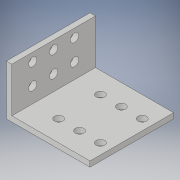
# Autodesk Inventor part: 2in bracket
Saved by Autodesk Inventor 2018 (Build 220112000, 112)
## iProperties
Created: 2020-01-25
Part Number: 2in bracket
Material: Generic
Document SubType Name: Modeling
Designer: s-2513225
Density: 1 g/cm^3
Appearance: Default
Author: s-2513225
Autodesk Inventor part; units mm, degrees
ref_plane "YZ Plane" through (0, 0, 0) normal (1, 0, 0) x (0, 1, 0)
ref_plane "XZ Plane" through (0, 0, 0) normal (0, 1, 0) x (-1, 0, 0)
ref_plane "XY Plane" through (0, 0, 0) normal (0, 0, 1) x (1, 0, 0)
sketch "Sketch1" plane through (0, 0, 0) normal (0, 0, 1) x (1, 0, 0)
  line L0 (0, 0) -> (50.8, 0)
  line L1 (50.8, 0) -> (50.8, 3.302)
  line L2 (50.8, 3.302) -> (3.302, 3.302)
  line L3 (0, 3.302) -> (0, 0)
  line L4 (3.302, 3.302) -> (3.302, 50.8)
  line L5 (3.302, 50.8) -> (0, 50.8)
  line L6 (0, 50.8) -> (0, 3.302)
  dimension "d1" = 3.302
  dimension "d2" = 3.302
  constraints: 14 end point, 3 parallel, 1 horizontal, 1 perpendicular
  measures "d1" distance of L1.end L0.end
  measures "d2" distance of L5.end L4.end
extrude "Extrusion1" add sketch "Sketch1" along normal blind 50.8
sketch "Sketch2" plane through (0, 0, 50.8) normal (0, 0, 1) x (1, 0, 0)
  line L0 (3.302, 50.8) -> (0, 50.8) construction
  line L1 (0, 50.8) -> (0, 30.48) construction
  line L2 (0, 50.8) -> (0, 0) construction
  line L3 (0, 30.48) -> (6.2781, 30.48)
  line L4 (6.2781, 30.48) -> (6.2781, 52.9453)
  line L5 (6.2781, 52.9453) -> (0, 52.9453)
  line L6 (0, 52.9453) -> (0, 30.48)
  line L7 (3.302, 3.302) -> (3.302, 50.8) construction
  line L8 (3.302, 30.48) -> (3.302, 0) construction
  dimension "d6" = 20.32
  dimension "d49" = 30.48
  constraints: 12 end point, 3 point on line, 2 parallel, 1 collinear, 1 horizontal, 1 perpendicular
  measures "d6" distance of L0.end L1.end
  measures "d49" distance of L8.start L8.end
extrude "Extrusion2" cut sketch "Sketch2" against normal blind 50.8
sketch "Sketch3" plane through (0, 0, 0) normal (-1, 0, 0) x (0, 0, 1)
  line L0 (0, 0) -> (50.8, 0) construction
  line L1 (0, 0) -> (12.7, 0) construction
  line L2 (12.7, 0) -> (25.4, 0) construction
  line L3 (25.4, 0) -> (38.1, 0) construction
  line L4 (38.1, 0) -> (38.1, 12.7) construction
  line L5 (38.1, 12.7) -> (38.1, 25.4) construction
  line L6 (25.4, 0) -> (25.4, 12.7) construction
  line L7 (25.4, 12.7) -> (25.4, 25.4) construction
  line L8 (12.7, 0) -> (12.7, 12.7) construction
  line L9 (12.7, 12.7) -> (12.7, 25.4) construction
  circle A0 centre (12.7, 25.4) radius 2.5797
  circle A1 centre (25.4, 25.4) radius 2.5797
  circle A2 centre (38.1, 25.4) radius 2.5797
  circle A3 centre (38.1, 12.7) radius 2.5797
  circle A4 centre (25.4, 12.7) radius 2.5797
  circle A5 centre (12.7, 12.7) radius 2.5797
  dimension "d9" = 12.7
  dimension "d10" = 12.7
  dimension "d11" = 12.7
  dimension "d12" = 12.7
  dimension "d13" = 12.7
  dimension "d14" = 12.7
  dimension "d15" = 12.7
  dimension "d16" = 12.7
  dimension "d17" = 12.7
  dimension "d18" = 5.1594
  dimension "d19" = 5.1594
  dimension "d20" = 5.1594
  dimension "d21" = 5.1594
  dimension "d22" = 5.1594
  dimension "d23" = 5.1594
  constraints: 18 end point, 6 centre point, 6 coincident, 5 point on line, 3 perpendicular, 1 midpoint
  measures "d9" distance of L0.start L1.end
  measures "d10" distance of L1.end L2.end
  measures "d11" distance of L2.end L3.end
  measures "d12" distance of L3.end L4.end
  measures "d13" distance of L4.end L5.end
  measures "d14" distance of L2.end L6.end
  measures "d15" distance of L6.end L7.end
  measures "d16" distance of L1.end L8.end
  measures "d17" distance of L8.end L9.end
  measures "d18" diameter of A0
  measures "d19" diameter of A1
  measures "d20" diameter of A2
  measures "d21" diameter of A3
  measures "d22" diameter of A4
  measures "d23" diameter of A5
extrude "Extrusion3" cut sketch "Sketch3" against normal blind 50.8
sketch "Sketch4" plane through (0, 0, 0) normal (0, -1, 0) x (1, 0, 0)
  line L0 (50.8, 0) -> (50.8, 50.8) construction
  line L1 (50.8, 50.8) -> (50.8, 38.1) construction
  line L2 (50.8, 38.1) -> (44.45, 38.1) construction
  line L3 (44.45, 38.1) -> (31.75, 38.1) construction
  line L4 (31.75, 38.1) -> (19.05, 38.1) construction
  line L5 (19.05, 38.1) -> (6.35, 38.1) construction
  line L6 (50.8, 0) -> (50.8, 13.462) construction
  circle A0 centre (44.45, 38.1) radius 2.5797
  circle A1 centre (31.75, 38.1) radius 2.5797
  circle A2 centre (19.05, 38.1) radius 2.5797
  line L7 (50.8, 23.876) -> (50.8, 12.7) construction
  line L8 (50.8, 12.7) -> (44.45, 12.7) construction
  line L9 (44.45, 12.7) -> (31.75, 12.7) construction
  line L10 (31.75, 12.7) -> (19.05, 12.7) construction
  line L11 (19.05, 12.7) -> (6.35, 12.7) construction
  circle A3 centre (44.45, 12.7) radius 2.5797
  circle A4 centre (31.75, 12.7) radius 2.5797
  circle A5 centre (19.05, 12.7) radius 2.5797
  line L12 (50.8, 13.462) -> (44.45, 13.462) construction
  point P0 (0, 0)
  dimension "d26" = 12.7
  dimension "d27" = 6.35
  dimension "d28" = 12.7
  dimension "d29" = 12.7
  dimension "d30" = 12.7
  dimension "d31" = 13.462
  dimension "d32" = 5.1594
  dimension "d33" = 5.1594
  dimension "d34" = 5.1594
  dimension "d37" = 6.35
  dimension "d38" = 12.7
  dimension "d39" = 12.7
  dimension "d40" = 12.7
  dimension "d41" = 5.1594
  dimension "d42" = 5.1594
  dimension "d43" = 5.1594
  constraints: 24 end point, 8 point on line, 6 centre point, 6 coincident, 1 horizontal, 1 perpendicular
  measures "d26" distance of L0.end L1.end
  measures "d27" distance of L1.end L2.end
  measures "d28" distance of L2.end L3.end
  measures "d29" distance of L3.end L4.end
  measures "d30" distance of L4.end L5.end
  measures "d31" distance of L0.start L6.end
  measures "d32" diameter of A0
  measures "d33" diameter of A1
  measures "d34" diameter of A2
  measures "d37" distance of L7.end L9.start
  measures "d38" distance of L9.start L10.start
  measures "d39" distance of L10.start L10.end
  measures "d40" distance of L10.end L11.end
  measures "d41" diameter of A3
  measures "d42" diameter of A4
  measures "d43" diameter of A5
extrude "Extrusion5" cut sketch "Sketch4" against normal blind 50.8
body "Solid1"
